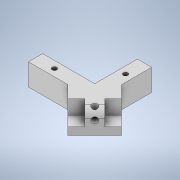
# Autodesk Inventor part: l_bracket
Saved by Autodesk Inventor 2021 (Build 250183000, 183)
## iProperties
Created: 2020-07-18
Part Number: l_bracket
Material: Generic
Document SubType Name: Modeling
Designer: Andrew
Density: 1 g/cm^3
Appearance: Default
Author: Andrew
Autodesk Inventor part; units mm, degrees
ref_plane "YZ Plane" through (0, 0, 0) normal (1, 0, 0) x (0, 1, 0)
sketch "Sketch1" plane through (0, 0, 0) normal (0, 1, 0) x (-1, 0, 0)
  line L0 (0, -70) -> (15, -70.0001)
  line L1 (15, -70.0001) -> (15.0003, -15.0001)
  line L2 (15.0003, -15.0001) -> (59.9999, -15.0004)
  line L3 (59.9999, -15.0004) -> (60, 0.0001)
  line L4 (60, 0.0001) -> (0, 0)
  line L5 (0, -70) -> (0, 0)
  dimension "d0" = 70
  dimension "d1" = 15
  dimension "d2" = 55
  dimension "d40" = 15.0005
  dimension "d41" = 60
  dimension "d42" = 44.9996
  constraints: 12 end point, 3 perpendicular, 1 vertical
  measures "d0" distance of L4.end L0.start
  measures "d1" distance of L0.start L0.end
  measures "d2" distance of L0.end L1.end
  measures "d40" distance of L2.end L3.end
  measures "d41" distance of L3.end L4.end
  measures "d42" distance of L1.end L2.end
extrude "Extrusion1" add sketch "Sketch1" along normal blind 23
sketch "Sketch2" plane through (0, 23, 0) normal (0, 1, 0) x (1, 0, 0)
  line L0 (0, 70) -> (-15, 70.0001) projected
  line L1 (0, 0) -> (0, 70) projected
  line L2 (-59.9999, 15.0004) -> (-60, -0.0001) projected
  line L3 (-60, -0.0001) -> (0, 0) projected
  point P0 (-7.5, 40)
  point P1 (-7.5, 60)
  point P2 (-30, 7.5)
  point P3 (-50, 7.4999)
  point P4 (0, 20)
  dimension "d14" = 10
  dimension "d15" = 30
  dimension "d16" = 7.5
  dimension "d17" = 7.5
  dimension "d18" = 10
  dimension "d19" = 30
  dimension "d20" = 7.5
  dimension "d21" = 7.5
  measures "d14" distance from line of L0 point (-7.5, 60)
  measures "d15" distance from line of L0 point (-7.5, 40)
  measures "d16" distance from line of L1 point (-7.5, 40)
  measures "d17" distance from line of L1 point (-7.5, 60)
  measures "d18" distance from line of L2 point (-50, 7.5)
  measures "d19" distance from line of L2 point (-30, 7.5)
  measures "d20" distance from line of L3 point (-50, 7.5)
  measures "d21" distance from line of L3 point (-30, 7.5)
hole "Hole1" at (-7.5, 23, -40) at (-7.5, 23, -60) at (-30, 23, -7.5) at (-50, 23, -7.4999) direction (0, -1, 0) diameter 4.134 depth 10 tip angle 118 thread size "M5x0.8" class "6H" standard "ANSI Metric M Profile"
sketch "Sketch3" plane through (0, 0, 0) normal (0, -1, 0) x (1, 0, 0)
  line L0 (0, -70) -> (-15, -70.0001) projected
  line L1 (0, 0) -> (0, -70) projected
  line L2 (-59.9999, -15.0004) -> (-60, 0.0001) projected
  line L3 (-60, 0.0001) -> (0, 0) projected
  point P0 (-7.5, -50)
  point P1 (-40, -7.4999)
  point P2 (0, -20)
  dimension "d29" = 20
  dimension "d30" = 7.5
  dimension "d31" = 20
  dimension "d32" = 7.5
  measures "d29" distance from line of L0 point (-7.5, -50)
  measures "d30" distance from line of L1 point (-7.5, -50)
  measures "d31" distance from line of L2 point (-40, -7.5)
  measures "d32" distance from line of L3 point (-40, -7.5)
hole "Hole2" at (-7.5, 0, -50) at (-40, 0, -7.4999) direction (0, 1, 0) diameter 4.917 depth 17.1 tip angle 118 thread size "M6x1" class "6H" standard "ANSI Metric M Profile"
sketch "Sketch4" plane through (0, 23, 0) normal (0, 1, 0) x (1, 0, 0)
  line L0 (-60, -0.0001) -> (0, 0) projected
  line L1 (23.5318, 4.7525) -> (0, 28.2843)
  line L2 (0, 28.2843) -> (-28.2842, 0)
  line L3 (-28.2842, 0) -> (-4.7524, -23.5318)
  line L4 (-4.7524, -23.5318) -> (23.5318, 4.7525)
  line L5 (0, 0) -> (0, 70) projected
  dimension "d180" = 40
  dimension "d181" = 33.279
  dimension "d182" = 45
  constraints: 8 end point, 2 parallel, 2 point on line, 1 perpendicular
  measures "d180" distance of L2.end L1.end
  measures "d181" distance of L1.start L1.end
  measures "d182" angle of L0 L3
ref_plane "Work Plane3" through (25, 0, -25) normal (-0.3535534, -0.8660254, -0.3535534) x (-0.7071068, 0, 0.7071068)
ref_plane "Work Plane4" through (25.5983, 25, -5.1859) normal (0.7071068, 0, 0.7071068) x (0.7071068, 0, -0.7071068)
extrude "Extrusion9" add sketch "Sketch4" against normal up to surface (23 mm away) contours L0 L5 L1 L4 L3
sketch "Sketch20" plane through (23.5318, 0, -4.7525) normal (0.7071079, 0, 0.7071057) x (0.7071057, 0, -0.7071079)
  line L0 (-12.5, 0) -> (-27.5, 0)
  line L1 (-27.5, 0) -> (-27.5, 15)
  line L2 (-27.5, 15) -> (-12.5, 15)
  line L3 (-12.5, 15) -> (-12.5, 0)
  line L4 (0, 23) -> (0, 0) projected
  line L5 (0, 0) -> (-40, 0) projected
  line L6 (-12.5, 15) -> (0, 15)
  line L7 (0, 15) -> (0, 0)
  line L8 (0, 0) -> (-12.5, 0)
  line L9 (-12.5, 0) -> (-12.5, 15)
  line L10 (-27.5, 15) -> (-40, 15)
  line L11 (-40, 15) -> (-40, 0)
  line L12 (-40, 0) -> (-27.5, 0)
  line L13 (-27.5, 0) -> (-27.5, 15)
  point P0 (-20, 0)
  dimension "d185" = 15
  dimension "d186" = 15
  dimension "d187" = 12.5
  constraints: 24 end point, 6 parallel, 3 horizontal, 3 perpendicular, 1 collinear
  measures "d185" distance of L1.end L2.end
  measures "d186" distance of L0.end L1.end
  measures "d187" distance between parallel lines of L4 L3
extrude "Extrusion14" cut sketch "Sketch20" against normal blind 15 contours L3 L6 L4 L5 | L5 L11 L10 L1
sketch "Sketch22" plane through (-4.7524, 0, 23.5318) normal (-0.7071057, 0, 0.7071079) x (0.7071079, 0, 0.7071057)
  line L0 (0, 0) -> (-33.279, 0) projected
  line L1 (0, 23) -> (0, 0) projected
  arc A0 (-7.5, 0) -> (0, 7.5) centre (-7.5, 7.5) ccw
  line L2 (-7.5, 0) -> (0, 0)
  line L3 (0, 7.5) -> (0, 0)
  point P0 (-13.279, 0)
  point P1 (-7.5, 7.5)
  dimension "d199" = 7.5
  dimension "d200" = 7.5
  constraints: 4 end point, 2 point on circle, 2 point on line, 2 tangent, 1 centre point, 1 collinear, 1 perpendicular
  measures "d199" distance of L2.start point (-7.5, 7.5)
  measures "d200" distance of point (-7.5, 7.5) L3.start
extrude "Extrusion16" cut sketch "Sketch22" against normal blind 40
sketch "Sketch23" plane through (23.5318, 15, -4.7525) normal (0.7071079, 0, 0.7071057) x (0.7071057, 0, -0.7071079)
  line L0 (-12.5, -15) -> (-27.5, -15) projected
  line L1 (-27.5, -7.5) -> (-27.5, -15) projected
  point P0 (-20, -15)
  point P1 (-20, -6)
  dimension "d201" = 9
  dimension "d202" = 7.5
  measures "d201" distance from line of L0 point (-20, -6)
  measures "d202" distance from line of L1 point (-20, -6)
hole "Hole5" at (9.3897, 9, 9.3897) direction (-0.7071079, 0, -0.7071057) diameter 6.2 depth 10 tip angle 118 clearance for "Flat Head Machine Screw" size "M6" standard "Ansi Metric M Profile"
sketch "Sketch24" plane through (0, 0, 0) normal (0, -1, 0) x (1, 0, 0)
  line L0 (7.4714, 11.308) -> (4.0864, 14.693) projected
  line L1 (4.0864, 14.693) -> (-1.2169, 9.3897) projected
  point P0 (0, 0)
  point P1 (5.1471, 5.147)
  dimension "d210" = 6
  dimension "d211" = 7.5
  measures "d210" distance from line of point (5.147, 5.147) L0
  measures "d211" distance from line of point (5.147, 5.147) L1
hole "Hole6" at (5.1471, 0, 5.147) direction (0, 1, 0) diameter 6.2 depth 10 tip angle 118 clearance for "Flat Head Machine Screw" size "M6" standard "Ansi Metric M Profile"
sketch "Sketch25" plane through (-6.5202, 0, 4.0864) normal (-0.7071057, 0, 0.7071079) x (0.7071079, 0, 0.7071057)
  line L0 (7.5, 0) -> (0, 0) projected
  line L1 (15, 15) -> (15, 7.5) projected
  point P0 (1.721, 0)
  point P1 (7.5, 7.5)
  dimension "d219" = 7.5
  dimension "d220" = 7.5
  measures "d219" distance from line of L0 point (7.5, 7.5)
  measures "d220" distance from line of L1 point (7.5, 7.5)
hole "Hole7" at (-1.2169, 7.5, 9.3897) direction (0.7071057, 0, -0.7071079) diameter 4.917 depth 4 thread size "M6x1" class "6H" standard "ISO Metric profile"
sketch "Sketch26" plane through (4.0864, 0, -6.5202) normal (0.7071057, 0, -0.7071079) x (-0.7071079, 0, -0.7071057)
  line L0 (0, 0) -> (-7.5, 0) projected
  line L1 (-15, 7.5) -> (-15, 15) projected
  point P0 (-1.721, 0)
  point P1 (-7.5, 7.5)
  dimension "d228" = 7.5
  dimension "d229" = 7.5
  measures "d228" distance from line of point (-7.5, 7.5) L0
  measures "d229" distance from line of L1 point (-7.5, 7.5)
hole "Hole8" at (9.3897, 7.5, -1.2169) direction (-0.7071057, 0, 0.7071079) diameter 4.917 depth 4 thread size "M6x1" class "6H" standard "ISO Metric profile"
body "Solid1"
